Autodesk Fusion 360 part; units mm, degrees
(part 2 of 2)
  constraint symmetric L1 L37.end L91.end
  constraint symmetric L1 L29.end L79.start
  constraint symmetric L1 L15.start L67.start
  constraint symmetric L1 L14.start L69.start
  constraint symmetric L1 A0 A45
  constraint symmetric L1 L15.end L67.end
  constraint symmetric L1 L16.start A39.end
  constraint symmetric L1 A1 A39
  constraint symmetric L1 L16.end A43.start
  constraint symmetric L1 L17.start L68.start
  constraint symmetric L1 A2 A43
  constraint symmetric L1 L17.end L68.end
  constraint symmetric L1 A3.start L69.end
  constraint symmetric L1 A3 A37
  constraint symmetric L1 L29.start L87.start
  constraint symmetric L1 L24.end L111.end
  constraint symmetric L1 L13.end L71.end
  constraint symmetric L1 L33.start L100.start
  constraint symmetric L1 L31.end L73.end
  constraint symmetric L1 L20.end L102.end
  constraint symmetric L1 L22.end A56.start
  constraint symmetric L1 A4 A56
  constraint symmetric L1 L19.end L70.end
  constraint symmetric L1 L21.start A36.start
  constraint symmetric L1 A5 A36
  constraint symmetric L1 L19.start L70.start
  constraint symmetric L1 L23.end L106.end
  constraint symmetric L1 A6 A54
  constraint symmetric L1 L20.start A46.end
  constraint symmetric L1 L21.end L78.end
  constraint symmetric L1 A7 A46
  constraint symmetric L1 L9.start A38.start
  constraint symmetric L1 L23.start A38.end
  constraint symmetric L1 A8 A38
  constraint symmetric L1 L12.start L105.start
  constraint symmetric L1 L9.end L83.end
  constraint symmetric L1 A9 A58
  constraint symmetric L1 L11.end A35.end
  constraint symmetric L1 L30.start A35.start
  constraint symmetric L1 A10 A35
  constraint symmetric L1 L25.end L74.end
  constraint symmetric L1 L26.start L81.start
  constraint symmetric L1 A11 A48
  constraint symmetric L1 L27.end L99.end
  constraint symmetric L1 L25.start L74.start
  constraint symmetric L1 A12 A52
  constraint symmetric L1 L13.start L71.start
  constraint symmetric L1 L27.start A47.end
  constraint symmetric L1 A13 A47
  constraint symmetric L1 L30.end L84.end
  constraint symmetric L1 L24.start L111.start
  constraint symmetric L1 A14 A57
  constraint symmetric L1 L28.end L75.start
  constraint symmetric L1 L26.end L81.end
  constraint symmetric L1 A15 A42
  constraint symmetric L1 L8.start A41.end
  constraint symmetric L1 L10.end L75.end
  constraint symmetric L1 A16 A41
  constraint symmetric L1 L31.start L73.start
  constraint symmetric L1 L43.start L119.start
  constraint symmetric L1 L47.start A63.end
  constraint symmetric L1 L39.end L108.end
  constraint symmetric L1 L43.end L119.end
  constraint symmetric L1 L35.end L131.end
  constraint symmetric L1 L40.start L76.start
  constraint symmetric L1 L47.end L130.end
  constraint symmetric L1 L54.start L120.start
  constraint symmetric L1 L36.start L128.start
  constraint symmetric L1 L49.end L72.end
  constraint symmetric L1 L40.end L76.end
  constraint symmetric L1 L45.end A67.end
  constraint symmetric L1 A21.end L101.start
  constraint symmetric L1 A22.end L72.start
  constraint symmetric L1 L42.end L98.end
  constraint symmetric L1 A17.start L89.start
  constraint symmetric L1 L48.start A51.end
  constraint symmetric L1 L45.start A62.start
  constraint symmetric L1 A17.end A53.start
  constraint symmetric L1 L38.start L90.start
  constraint symmetric L1 A24.start A62.end
  constraint symmetric L1 L44.start L80.start
  constraint symmetric L1 L41.end L82.end
  constraint symmetric L1 A18.start L101.end
  constraint symmetric L1 A18.end L125.end
  constraint symmetric L1 L51.start L94.start
  constraint symmetric L1 L46.end L126.end
  constraint symmetric L1 A20.end L104.end
  constraint symmetric L1 A28.end L77.end
  constraint symmetric L1 L35.start L131.start
  constraint symmetric L1 L36.end L128.end
  constraint symmetric L1 L37.start L127.start
  constraint symmetric L1 A17 A53
  constraint symmetric L1 L3.end L88.end
  constraint symmetric L1 A18 A68
  constraint symmetric L1 L4.start L82.start
  constraint symmetric L1 A19 A64
  constraint symmetric L1 L42.start A50.end
  constraint symmetric L1 L44.end L80.end
  constraint symmetric L1 A20 A61
  constraint symmetric L1 A21 A67
  constraint symmetric L1 A22 A55
  constraint symmetric L1 L39.start L108.start
  constraint symmetric L1 A23 A51
  constraint symmetric L1 A24 A62
  constraint symmetric L1 A25 A44
  constraint symmetric L1 A26 A63
  constraint symmetric L1 A27 A66
  constraint symmetric L1 A28 A50
  constraint symmetric L1 L57.start L77.start
  constraint symmetric L1 A29 A49
  constraint symmetric L1 L58.start A60.end
  constraint symmetric L1 L58.end L121.end
  constraint symmetric L1 A30 A65
  constraint symmetric L1 A31.end A60.start
  constraint symmetric L1 A31 A60
  constraint symmetric L1 A32.end A59.start
  constraint symmetric L1 A32.start A59.end
  constraint symmetric L1 A32 A59
  constraint symmetric L1 L59.start L129.start
  constraint symmetric L1 A33 A69
  constraint symmetric L1 L4.end L118.end
  constraint symmetric L1 A34.end A40.start
  constraint symmetric L1 A34 A40
  constraint symmetric L1 A34.start A40.end
  constraint symmetric L1 L14.end L85.end
  measures "d1" distance of L95.start L62.start
  measures "d5" distance of L2.start L2.end
  measures "d10" distance of L11 L12
  measures "d11" distance of L22 L23
  measures "d13" distance of L9 L16
  measures "d15" radius of A1
  measures "d16" radius of A2
  measures "d17" radius of A3
  measures "d19" radius of A4
  measures "d20" radius of A5
  measures "d21" radius of A6
  measures "d22" radius of A8
  measures "d23" radius of A9
  measures "d24" radius of A10
  measures "d25" radius of A11
  measures "d26" radius of A12
  measures "d27" radius of A13
  measures "d28" radius of A14
  measures "d29" radius of A15
  measures "d30" radius of A16
extrude "Extrude1" add sketch "Sketch1" along normal blind 3000
scale "Scale1" factor 0.1 about (-108.1058, 95, 0) bodies 1
scale "Scale2" factor 0.666667 about (-108.1058, 95, 0) bodies 1
equation "d5 = ( 85.3 / 2 ) * 1 mm"
equation "d34 = 1 / 1.5"
